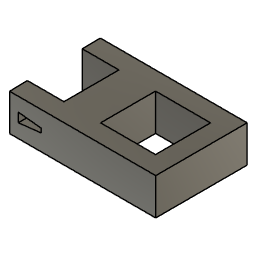
bottom part (Autodesk Fusion 360 design; units mm, degrees)
Autodesk Fusion 360 part; units mm, degrees
sketch "Sketch1" plane through (0, 0, 0) normal (0, 0, 1) x (1, 0, 0)
  line L0 (29.848, 60) -> (110, 60)
  line L1 (110, 60) -> (110, 10.0866)
  line L2 (110, 10.0866) -> (30.2597, 10.0866)
  line L3 (100, 50) -> (70, 50)
  line L4 (70, 50) -> (70, 20)
  line L5 (70, 20) -> (100, 20)
  line L6 (100, 20) -> (100, 50)
  line L7 (30, 50) -> (50, 50)
  line L8 (50, 50) -> (50, 20)
  line L9 (50, 20) -> (30, 20)
  line L10 (29.848, 60) -> (30, 50)
  line L11 (30, 20) -> (30.2597, 10.0866)
  constraint horizontal L0
  constraint vertical L1
  constraint horizontal L2
  constraint horizontal L3
  constraint vertical L4
  constraint horizontal L5
  constraint vertical L6
  constraint horizontal L7
  constraint vertical L8
  constraint horizontal L9
extrude "Extrude1" add sketch "Sketch1" along normal blind 20
sketch "Sketch2" plane through (0, 10.0866, 0) normal (0, -1, 0) x (1, 0, 0)
  line L0 (30.2597, 0) -> (110, 0)
  line L1 (110, 0) -> (110, 20)
  line L2 (110, 20) -> (30.2597, 20)
  line L3 (30.2597, 20) -> (30.2597, 0)
  line L4 (47.5008, 8.9134) -> (47.5008, 11.176)
  line L5 (35, 12.5) -> (35, 7.5)
  line L6 (35, 7.5) -> (47.5008, 8.9134)
  line L7 (35, 12.5) -> (47.5008, 11.176)
  line L8 (47.6079, 8.9255) -> (47.5008, 9.8724)
  constraint vertical L4
  constraint vertical L5
  constraint coincident L6 L8.start
  constraint perpendicular L6 L8
  constraint coincident L4 L8.end
extrude "Extrude2" cut sketch "Sketch2" against normal blind 11 contours L4 L5 L6 L7
